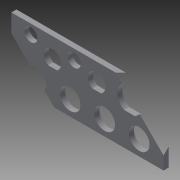
# Autodesk Inventor part: Yagi_Front_BackPlate
Saved by Autodesk Inventor 2014 (Build 180170000, 170)
## iProperties
Created: 2015-01-07
Part Number: Yagi_Front_BackPlate
Material: Generic
Document SubType Name: Modeling
Designer: Owner
Density: 1 g/cm^3
Appearance: Default
Author: Owner
Autodesk Inventor part; units mm, degrees
ref_plane "YZ Plane" through (0, 0, 0) normal (1, 0, 0) x (0, 1, 0)
ref_plane "XZ Plane" through (0, 0, 0) normal (0, 1, 0) x (-1, 0, 0)
ref_plane "XY Plane" through (0, 0, 0) normal (0, 0, 1) x (1, 0, 0)
sketch "Sketch1" plane through (0, 0, 0) normal (0, 0, 1) x (1, 0, 0)
  line L0 (-43.8846, -36.7982) -> (51.3654, -36.7982)
  line L1 (51.3654, -36.7982) -> (51.3654, -87.5982)
  line L2 (51.3654, -87.5982) -> (-43.8846, -87.5982)
  line L3 (-43.8846, -87.5982) -> (-43.8846, -36.7982)
  point P0 (0, 0)
  dimension "d0" = 95.25
  dimension "d1" = 50.8
  constraints: 8 end point, 2 parallel, 1 horizontal, 1 perpendicular
  measures "d0" distance of L0.start L0.end
  measures "d1" distance of L0.end L1.end
extrude "Extrusion1" add sketch "Sketch1" along normal blind 3.175
sketch "Sketch2" plane through (0, 0, 0) normal (0, 0, -1) x (-1, 0, 0)
  line L0 (-51.3654, -36.7982) -> (-51.3654, -87.5982) projected
  line L1 (43.8846, -87.5982) -> (43.8846, -36.7982) projected
  circle A0 centre (-36.1254, -74.8982) radius 6.477
  circle A1 centre (-14.5354, -74.8982) radius 6.477
  circle A2 centre (28.6446, -74.8982) radius 6.477
  circle A3 centre (7.0546, -74.8982) radius 6.477
  line L2 (-51.3654, -87.5982) -> (43.8846, -87.5982) projected
  circle A4 centre (-10.7168, -56.969) radius 9.0932 construction
  arc A5 (-7.9777, -61.6934) -> (-13.4559, -61.6934) centre (-10.7168, -56.969) ccw
  line L3 (-13.4559, -61.6934) -> (-7.9777, -61.6934)
  circle A6 centre (-31.2509, -56.402) radius 10.3124 construction
  arc A7 (-28.0085, -63.4378) -> (-34.4934, -63.4378) centre (-31.2509, -56.402) ccw
  line L4 (-34.4934, -63.4378) -> (-28.0085, -63.4378)
  circle A8 centre (16.927, -58.2867) radius 9.0932 construction
  arc A9 (19.6661, -63.0111) -> (14.1879, -63.0111) centre (16.927, -58.2867) ccw
  line L5 (14.1879, -63.0111) -> (19.6661, -63.0111)
  circle A10 centre (30.5118, -51.8427) radius 4.1
  circle A11 centre (30.5118, -51.8427) radius 5.25 construction
  circle A12 centre (3.3593, -52.1547) radius 4.1
  circle A13 centre (3.3593, -52.1547) radius 5.25 construction
  line L6 (43.8846, -54.5366) -> (43.8846, -40.5212)
  point P0 (0, 0)
  dimension "d4" = 12.954
  dimension "d5" = 12.954
  dimension "d6" = 12.954
  dimension "d7" = 12.954
  dimension "d8" = 15.24
  dimension "d11" = 15.24
  dimension "d12" = 21.59
  dimension "d14" = 21.59
  dimension "d18" = 12.7
  dimension "d19" = 12.7
  dimension "d20" = 12.7
  dimension "d21" = 12.7
  dimension "d28" = 18.1864
  dimension "d29" = 10.922
  dimension "d30" = 4.7244
  dimension "d31" = 20.6248
  dimension "d32" = 15.494
  dimension "d33" = 7.0358
  dimension "d34" = 18.1864
  dimension "d35" = 10.922
  dimension "d36" = 4.7244
  dimension "d37" = 8.2
  dimension "d38" = 10.5
  dimension "d41" = 8.2
  dimension "d42" = 10.5
  constraints: 14 centre point, 8 end point, 6 point on circle, 5 coincident, 1 parallel, 1 point on line
  measures "d4" diameter of A2
  measures "d5" diameter of A3
  measures "d6" diameter of A1
  measures "d7" diameter of A0
  measures "d8" distance from line of L1 A2.centre
  measures "d11" distance from line of L0 A0.centre
  measures "d12" distance of A1.centre A0.centre
  measures "d14" distance of A2.centre A3.centre
  measures "d18" distance from line of L2 A0.centre
  measures "d19" distance from line of L2 A1.centre
  measures "d20" distance from line of L2 A3.centre
  measures "d21" distance from line of L2 A2.centre
  measures "d28" diameter of A4
  measures "d29" diameter of A5
  measures "d30" distance from line of L3 A5.centre
  measures "d31" diameter of A6
  measures "d32" diameter of A7
  measures "d33" distance from line of A7.centre L4
  measures "d34" diameter of A8
  measures "d35" diameter of A9
  measures "d36" distance from line of L5 A9.centre
  measures "d37" diameter of A10
  measures "d38" diameter of A11
  measures "d41" diameter of A12
  measures "d42" diameter of A13
extrude "Extrusion2" cut sketch "Sketch2" against normal blind 6.35
body "Solid1"
